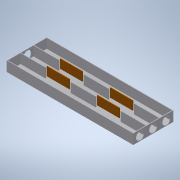
# Autodesk Inventor part: Distribuidor de truchas
Saved by Autodesk Inventor 2020 (Build 240168000, 168)
## iProperties
Created: 2020-02-23
Part Number: Distribuidor de truchas
Material: Plástico ABS
Document SubType Name: Modeling
Designer: PabloGod
Density: 1.06 g/cm^3
Appearance: Suave - Blanco
Mass: 2419.33 g
Surface Area: 9259.88 cm^2
Volume: 2282.38 cm^3
Author: PabloGod
Autodesk Inventor part; units mm, degrees
ref_plane "YZ Plane" through (0, 0, 0) normal (1, 0, 0) x (0, 1, 0)
ref_plane "XZ Plane" through (0, 0, 0) normal (0, 1, 0) x (-1, 0, 0)
sketch "Boceto1" plane through (0, 0, 0) normal (0, 1, 0) x (-1, 0, 0)
  line L0 (0, 0) -> (300, 0)
  line L1 (300, 0) -> (300, -320)
  line L2 (300, -320) -> (-710, -320)
  line L3 (0, 0) -> (-400, 0)
  line L4 (-400, 0) -> (-710, 0)
  line L5 (-710, 0) -> (-710, -320)
  line L6 (300, -105) -> (-710, -105)
  line L7 (300, -110) -> (-710, -110)
  line L8 (300, -210) -> (-710, -210)
  line L9 (300, -215) -> (-710, -215)
  line L10 (295, 0) -> (295, -320)
  line L11 (-705, 0) -> (-705, -320)
  line L12 (300, -5) -> (-710, -5)
  line L13 (300, -315) -> (-710, -315)
  point P0 (300, -147.5)
  point P1 (295, -105)
  point P2 (-705, -105)
  point P3 (-705, -5)
  point P4 (295, -5)
  point P5 (295, -215)
  point P6 (295, -315)
  point P7 (-705, -315)
  point P8 (-705, -215)
  point P9 (295, -110)
  point P10 (295, -210)
  point P11 (-705, -210)
  point P12 (-705, -110)
  dimension "d6" = 100
  dimension "d7" = 37.5
  dimension "d9" = 5
  dimension "d10" = 5
  dimension "d14" = 5
  dimension "d15" = 5
  dimension "d16" = 5
  dimension "d17" = 5
  dimension "d38" = 100
  dimension "d39" = 100
  dimension "d59" = 1010
  constraints: 26 end point, 11 point on line, 3 horizontal, 3 perpendicular, 1 coincident, 10 other
  measures "d6" distance of L7.start L8.start
  measures "d7" distance of L7.start point (300, -147.5)
  measures "d9" distance of L6.start L7.start
  measures "d10" distance of L8.start L9.start
  measures "d14" distance of L10.start L0.end
  measures "d15" distance of L4.end L11.start
  measures "d16" distance of point (300, 0) L12.start
  measures "d17" distance of L2.start L13.start
  measures "d38" distance of L12.start L6.start
  measures "d39" distance of L9.start L13.start
extrude "Extrusión1" add sketch "Boceto1" against normal blind 75 contours L0 L10 L12 L11 L4 L3 | L0 L1 L12 L10 | L12 L1 L6 L10 | L11 L12 L5 L4 | L10 L7 L11 L6 | L6 L1 L7 L10 | L11 L6 L5 L12 | L11 L7 L5 L6 | L7 L1 L8 L10 | L11 L8 L5 L7 | L10 L9 L11 L8 | L8 L1 L9 L10 | L11 L9 L5 L8 | L9 L1 L13 L10 | L11 L13 L5 L9 | L13 L1 L2 L10 | L10 L2 L11 L13 | L11 L2 L5 L13
sketch "Boceto2" plane through (0, -75, 0) normal (0, -1, 0) x (1, 0, 0)
  line L0 (710, -320) -> (710, 0) projected
  line L1 (710, -320) -> (-300, -320)
  line L2 (-300, -320) -> (-300, 0)
  line L3 (-300, 0) -> (710, 0)
  line L4 (710, 0) -> (710, -320)
  point P0 (0, 0)
  point P1 (710, 0)
  constraints: 8 end point, 2 parallel, 1 horizontal, 1 perpendicular
extrude "Extrusión2" add sketch "Boceto2" along normal blind 5
sketch "Boceto5" plane through (710, 0, 0) normal (1, 0, 0) x (0, 0, -1)
  line L0 (0, 0) -> (0, -80) projected
  line L1 (320, 0) -> (0, 0) projected
  line L2 (0, -80) -> (320, -80) projected
  circle A0 centre (160, -42.5) radius 32.5
  circle A1 centre (265, -42.5) radius 32.5
  circle A2 centre (55, -42.5) radius 32.5
  line L3 (55, 0) -> (55, -80)
  line L4 (320, -80) -> (0, -80) projected
  line L5 (160, 0) -> (160, -80)
  line L6 (265, 0) -> (265, -80)
  point P0 (0, 0)
  point P1 (5, 0)
  point P2 (105, 0)
  point P3 (110, 0)
  point P4 (210, 0)
  point P5 (215, 0)
  point P6 (315, 0)
  dimension "d40" = 5
  dimension "d41" = 5
  dimension "d42" = 5
  dimension "d43" = 5
  dimension "d44" = 100
  dimension "d45" = 100
  dimension "d46" = 50
  dimension "d47" = 65
  dimension "d48" = 50
  dimension "d49" = 65
  dimension "d50" = 50
  dimension "d51" = 65
  dimension "d52" = 37.5
  dimension "d53" = 37.5
  dimension "d54" = 37.5
  constraints: 6 end point, 3 centre point, 2 coincident, 2 perpendicular, 2 point on line, 1 midpoint, 10 other
  measures "d40" distance of point (315, 0) point (320, 0)
  measures "d41" distance of point (210, 0) point (215, 0)
  measures "d42" distance of point (110, 0) point (105, 0)
  measures "d43" distance of point (0, 0) point (5, 0)
  measures "d44" distance of point (5, 0) point (105, 0)
  measures "d45" distance of point (110, 0) point (210, 0)
  measures "d46" distance of point (110, 0) L5.start
  measures "d47" diameter of A0
  measures "d48" distance of point (215, 0) L6.start
  measures "d49" diameter of A1
  measures "d50" distance of point (5, 0) L3.start
  measures "d51" diameter of A2
  measures "d52" distance of L3.end A2.centre
  measures "d53" distance of L5.end A0.centre
  measures "d54" distance of L6.end A1.centre
extrude "Extrusión4" cut sketch "Boceto5" against normal blind 75 contours L3 A2 | A2 L3 | L6 A1 | A1 L6
extrude "Extrusión5" cut sketch "Boceto5" against normal through all contours L5 A0 | A0 L5
sketch "Boceto7" plane through (0, 0, 0) normal (0, 1, 0) x (1, 0, 0)
  line L0 (710, 320) -> (-300, 320) projected
  line L1 (-300, 320) -> (-300, 0) projected
  line L2 (-300, 0) -> (710, 0) projected
  line L3 (710, 0) -> (710, 320) projected
  line L4 (705, 105) -> (705, 5) projected
  line L5 (705, 5) -> (-295, 5) projected
  line L6 (-295, 5) -> (-295, 105) projected
  line L7 (-295, 105) -> (705, 105) projected
  line L8 (705, 315) -> (705, 215) projected
  line L9 (705, 215) -> (-295, 215) projected
  line L10 (-295, 215) -> (-295, 315) projected
  line L11 (-295, 315) -> (705, 315) projected
  line L12 (-295, 210) -> (705, 210) projected
  line L13 (705, 210) -> (705, 110) projected
  line L14 (705, 110) -> (-295, 110) projected
  line L15 (-295, 110) -> (-295, 210) projected
  line L16 (-295, 105) -> (705, 105) projected
  line L17 (-95, 105) -> (105, 105)
  line L18 (105, 105) -> (105, 110)
  line L19 (105, 110) -> (-95, 110)
  line L20 (-95, 110) -> (-95, 105)
  line L21 (705, 110) -> (-295, 110) projected
  line L22 (305, 105) -> (505, 105)
  line L23 (505, 105) -> (505, 110)
  line L24 (505, 110) -> (305, 110)
  line L25 (305, 110) -> (305, 105)
  line L26 (-295, 210) -> (705, 210) projected
  line L27 (-295, 215) -> (705, 215) projected
  line L28 (505, 210) -> (305, 210)
  line L29 (305, 210) -> (305, 215)
  line L30 (305, 215) -> (505, 215)
  line L31 (505, 215) -> (505, 210)
  line L32 (105, 210) -> (-95, 210)
  line L33 (-95, 210) -> (-95, 215)
  line L34 (-95, 215) -> (105, 215)
  line L35 (105, 215) -> (105, 210)
  point P0 (0, 0)
  point P1 (105, 105)
  point P2 (505, 105)
  point P3 (-95, 210)
  point P4 (305, 210)
  dimension "d86" = 200
  dimension "d87" = 200
  dimension "d88" = 200
  dimension "d89" = 200
  dimension "d90" = 200
  dimension "d91" = 200
  dimension "d92" = 200
  dimension "d93" = 200
  constraints: 32 end point, 12 point on line, 8 parallel, 4 horizontal, 4 perpendicular, 2 coincident
  measures "d86" distance of L17.start point (-295, 105)
  measures "d87" distance of point (105, 105) L17.start
  measures "d88" distance of L22.start point (105, 105)
  measures "d89" distance of point (505, 105) L22.start
  measures "d90" distance of point (-95, 210) point (-295, 210)
  measures "d91" distance of L32.start point (-95, 210)
  measures "d92" distance of point (305, 210) L32.start
  measures "d93" distance of L28.start point (305, 210)
extrude "Extrusión7" cut sketch "Boceto7" against normal blind 75 contours L7 L25 L14 L23 | L7 L20 L14 L18 | L12 L29 L9 L31 | L12 L33 L9 L35
ref_plane "Plano de trabajo1" through (0, -55, 0) normal (0, 1, 0) x (1, 0, 0)
sketch "Boceto11" plane through (0, -55, 0) normal (0, 1, 0) x (1, 0, 0)
  line L0 (305, 210) -> (105, 210) projected
  line L1 (105, 215) -> (105, 210) projected
  line L2 (105, 215) -> (305, 215) projected
  line L3 (305, 210) -> (305, 215) projected
  line L4 (305, 105) -> (105, 105) projected
  line L5 (105, 110) -> (105, 105) projected
  line L6 (105, 110) -> (305, 110) projected
  line L7 (305, 105) -> (305, 110) projected
  line L8 (505, 215) -> (505, 210) projected
  line L9 (505, 215) -> (705, 215) projected
  line L10 (705, 215) -> (705, 265) projected
  line L11 (705, 265) -> (705, 315) projected
  line L12 (705, 315) -> (-295, 315) projected
  line L13 (-295, 315) -> (-295, 215) projected
  line L14 (-295, 215) -> (-95, 215) projected
  line L15 (-95, 210) -> (-95, 215) projected
  line L16 (-95, 210) -> (-295, 210) projected
  line L17 (-295, 210) -> (-295, 160) projected
  line L18 (-295, 160) -> (-295, 110) projected
  line L19 (-295, 110) -> (-95, 110) projected
  line L20 (-95, 105) -> (-95, 110) projected
  line L21 (-95, 105) -> (-295, 105) projected
  line L22 (-295, 105) -> (-295, 5) projected
  line L23 (-295, 5) -> (705, 5) projected
  line L24 (705, 5) -> (705, 55) projected
  line L25 (705, 55) -> (705, 105) projected
  line L26 (705, 105) -> (505, 105) projected
  line L27 (505, 110) -> (505, 105) projected
  line L28 (505, 110) -> (705, 110) projected
  line L29 (705, 110) -> (705, 160) projected
  line L30 (705, 160) -> (705, 210) projected
  line L31 (705, 210) -> (505, 210) projected
  line L32 (105, 210) -> (305, 210) projected
  line L33 (705, 105) -> (505, 105) projected
  line L34 (305, 105) -> (105, 105) projected
  line L35 (-85, 210) -> (95, 210)
  line L36 (95, 210) -> (95, 215)
  line L37 (95, 215) -> (-85, 215)
  line L38 (-85, 215) -> (-85, 210)
  line L39 (-85, 105) -> (95, 105)
  line L40 (95, 105) -> (95, 110)
  line L41 (95, 110) -> (-85, 110)
  line L42 (-85, 110) -> (-85, 105)
  line L43 (315, 105) -> (495, 105)
  line L44 (495, 105) -> (495, 110)
  line L45 (495, 110) -> (315, 110)
  line L46 (315, 110) -> (315, 105)
  line L47 (315, 210) -> (495, 210)
  line L48 (495, 210) -> (495, 215)
  line L49 (495, 215) -> (315, 215)
  line L50 (315, 215) -> (315, 210)
  point P0 (0, 0)
  point P1 (495, 210)
  dimension "d113" = 10
  dimension "d114" = 10
  dimension "d115" = 10
  dimension "d116" = 10
  dimension "d117" = 10
  dimension "d118" = 10
  dimension "d119" = 10
  dimension "d120" = 10
  constraints: 32 end point, 8 coincident, 8 parallel, 4 horizontal, 4 perpendicular, 4 point on line
  measures "d113" distance of point (-95, 210) L35.start
  measures "d114" distance of point (-95, 105) L39.start
  measures "d115" distance of point (105, 105) point (95, 105)
  measures "d116" distance of point (105, 210) point (95, 210)
  measures "d117" distance of L47.start point (305, 210)
  measures "d118" distance of L43.start point (305, 105)
  measures "d119" distance of point (495, 105) point (505, 105)
  measures "d120" distance of point (505, 210) point (495, 210)
extrude "Extrusión8" add sketch "Boceto11" along normal blind 70 contours L38 L37 L36 L35 | L42 L41 L40 L39 | L46 L45 L44 L43 | L50 L49 L48 L47
